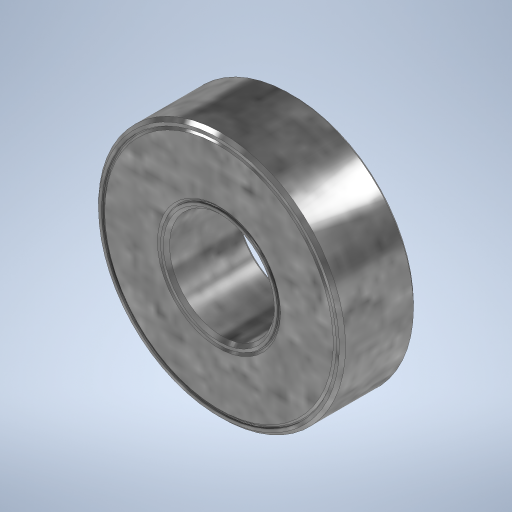
# Autodesk Inventor part: 6203베어링
Saved by Autodesk Inventor 2023 (Build 270158000, 158)
## iProperties
Created: 2022-06-08
Part Number: 6203베어링
Material: 일반
Document SubType Name: Modeling
Designer: fly01
Density: 1 g/cm^3
Appearance: 기본값
Author: fly01
Autodesk Inventor part; units mm, degrees
ref_plane "YZ Plane" through (0, 0, 0) normal (1, 0, 0) x (0, 1, 0)
ref_plane "XZ Plane" through (0, 0, 0) normal (0, 1, 0) x (-1, 0, 0)
ref_plane "XY Plane" through (0, 0, 0) normal (0, 0, 1) x (1, 0, 0)
sketch "스케치1" plane through (0, 0, 0) normal (0, 0, 1) x (1, 0, 0)
  circle A0 centre (0, 0) radius 8.5
  circle A1 centre (0, 0) radius 20
  dimension "d0" = 17
  dimension "d1" = 40
  constraints: 2 centre point, 2 coincident
  measures "d0" diameter of A0
  measures "d1" diameter of A1
extrude "돌출1" add sketch "스케치1" along normal mid plane 12
chamfer "모따기1" distance 0.5 angle 45 4 edges at (-20, 0, 6) (-20, 0, -6) (-8.5, 0, 6) (-8.5, 0, -6)
sketch "스케치2" plane through (0, 0, 0) normal (0, 1, 0) x (-1, 0, 0)
  line L0 (-19.5, 6) -> (19.5, 6) projected
  line L1 (19, 6) -> (19, 5.7414)
  line L2 (18.8293, 5.6707) -> (18.5, 6)
  line L3 (19.9584, 0) -> (8.5, 0)
  line L4 (8.5, 5.5) -> (8.5, -5.5) projected
  arc A0 (18.8293, 5.6707) -> (19, 5.7414) centre (18.9, 5.7414) ccw
  line L5 (14.2292, 0) -> (14.2292, 1.7292)
  line L6 (9.4584, 6) -> (9.4584, 5.7414)
  line L7 (9.6291, 5.6707) -> (9.9584, 6)
  arc A1 (9.4584, 5.7414) -> (9.6291, 5.6707) centre (9.5584, 5.7414) ccw
  line L8 (19, -6) -> (19, -5.7414)
  line L9 (18.8293, -5.6707) -> (18.5, -6)
  arc A2 (19, -5.7414) -> (18.8293, -5.6707) centre (18.9, -5.7414) ccw
  line L10 (9.4584, -6) -> (9.4584, -5.7414)
  line L11 (9.6291, -5.6707) -> (9.9584, -6)
  arc A3 (9.6291, -5.6707) -> (9.4584, -5.7414) centre (9.5584, -5.7414) ccw
  line L12 (0, 0) -> (0, -13.1586)
  line L13 (19.5, -6) -> (-19.5, -6) projected
  point P0 (19, 5.5)
  point P1 (8.9584, 6)
  point P2 (9.4584, 5.5)
  point P3 (19, -5.5)
  point P4 (8.9584, -6)
  point P5 (9.4584, -5.5)
  dimension "d7" = 0.5
  dimension "d8" = 0.5
  dimension "d9" = 0.5
  dimension "d10" = 0.1
  constraints: 22 end point, 21 symmetric about line, 10 point on line, 8 point on circle, 4 centre point, 3 vertical, 2 midpoint, 2 tangent, 3 other
  measures "d7" distance of L0.end L1.start
  measures "d8" distance of L1.start point (19, 5.5)
  measures "d9" distance of L1.start L2.end
  measures "d10" radius of A0
revolve "회전1" cut sketch "스케치2" angle 360 about axis through (0, 0, 0) along (0, 0, -1)
